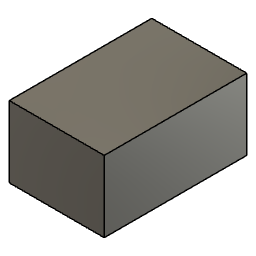
Create 5 (Autodesk Fusion 360 design; units mm, degrees)
Autodesk Fusion 360 part; units mm, degrees
box "BoxPrimitive1" add length 120 width 80 height 60 placed x (0, 0, -1) y (-1, 0, 0) z (0, 1, 0) at (80, 0, 0)
shell "Shell1" thickness 5 removed faces 1 at (26.6667, 0, -40)
sketch "Sketch2" plane through (0, 0, 0) normal (0, -1, 0) x (1, 0, 0)
  line L0 (75, -5) -> (75, -115)
  line L1 (75, -115) -> (5, -115)
  line L2 (5, -115) -> (5, -5)
  line L3 (5, -5) -> (75, -5)
  line L4 (0, -120) -> (80, -120)
  line L5 (80, -120) -> (80, 0)
  line L6 (80, 0) -> (0, 0)
  line L7 (0, 0) -> (0, -120)
  line L8 (5, -115) -> (75, -115)
  line L9 (75, -115) -> (75, -5)
  line L10 (75, -5) -> (5, -5)
  line L11 (5, -5) -> (5, -115)
  line L12 (5, -5) -> (75, -115)
  line L13 (75, -5) -> (5, -115)
  line L14 (40, -60) -> (40, -5)
  line L15 (40, -60) -> (40, -115)
  line L16 (40, -60) -> (75, -60)
  line L17 (40, -60) -> (5, -60)
  constraint coincident L2.end L3.start
  constraint coincident L0.end L1.start
  constraint coincident L0.start L3.end
  constraint coincident L1.end L2.start
  constraint midpoint L13 L14.start
  constraint midpoint L10 L14.end
  constraint midpoint L1 L15.end
  constraint midpoint L9 L16.end
  constraint midpoint L2 L17.end
ref_plane "WorkPlane1" through (40, 30, -60) normal (1, 0, 0) x (0, -1, 0)
sketch "Sketch3" plane through (40, 30, -60) normal (1, 0, 0) x (0, 0, -1)
  line L0 (-30, 70) -> (20, 70)
  line L1 (20, 70) -> (60, 30)
  line L2 (-30, 70) -> (-60, 30)
  constraint horizontal L0
